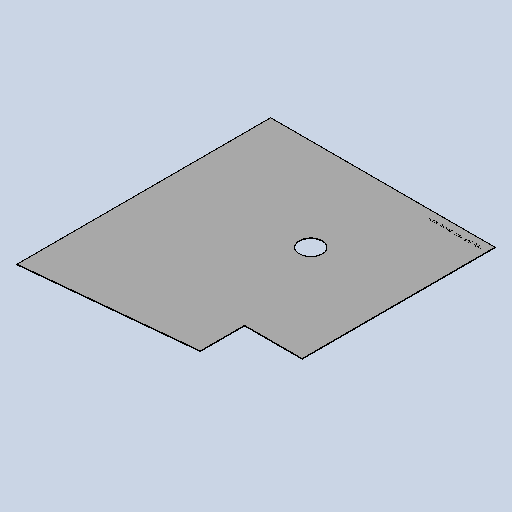
# Autodesk Inventor part: TRM 016 right board main+
Saved by Autodesk Inventor 2025 (Build 290162010, 162A)
## iProperties
Created: 2024-08-07
Part Number: TRM 016 right board main+
Material: AISI 304
Document SubType Name: Sheet Metal
Designer: pokla
Stock Number: ТРМ 015 левый борт основное
Density: 8.02768 g/cm^3
Flat Pattern Width: 77.93 cm
Flat Pattern Length: 88.1266 cm
Flat Pattern Area: 6867.71 cm^2
Sheet Metal Rule: AISI304 2mm Die16
Sheet Metal Width: 779,300 mm
Sheet Metal Length: 881,266 mm
Sheet Metal Area: 686770,668 mm^2
Appearance: Default
Author: pokla
Autodesk Inventor part; units mm, degrees
ref_plane "YZ Plane" through (0, 0, 0) normal (1, 0, 0) x (0, 1, 0)
ref_plane "XZ Plane" through (0, 0, 0) normal (0, 1, 0) x (-1, 0, 0)
ref_plane "XY Plane" through (0, 0, 0) normal (0, 0, 1) x (1, 0, 0)
sketch "Sketch1" plane through (0, 0, 0) normal (0, 0, 1) x (1, 0, 0)
  line L0 (-459.3004, -153.7378) -> (320, -153.7378)
  line L1 (320, -153.7378) -> (320, 670)
  line L2 (320, 670) -> (-459.3004, 670)
  line L3 (-459.3004, 670) -> (-459.3004, -153.7378)
  line L4 (120, -153.7378) -> (320, 0)
  circle A0 centre (0, 350) radius 40
  line L5 (320, 0) -> (120, 0)
  line L6 (120, 0) -> (120, -153.7378)
  line L7 (-459.3004, -153.7378) -> (-459.3004, -211.2657)
  line L8 (-459.3004, -211.2657) -> (120, -153.7378)
  point P0 (0, 0)
  dimension "d14" = 80
  dimension "d15" = 320
  dimension "d16" = 200
  dimension "d17" = 320
  dimension "d18" = 350
  measures "d14" diameter of A0
  measures "d15" distance from line of A0.centre L2
  measures "d16" distance of L4.end L5.end
  measures "d17" distance from line of L1 A0.centre
  measures "d18" distance of point (0, 0) A0.centre
extrude "Plate1" add sketch "Sketch1" along normal blind 2 contours L3 L2 L1 L5 L6 L0 | L0 L8 L7
sketch "Sketch2" plane through (0, 0, 0) normal (0, 0, -1) x (-1, 0, 0)
  line L0 (-300, 650) -> (-100, 650) construction
  line L1 (-100, 650) -> (-100, 630) construction
  line L2 (-100, 630) -> (-300, 630) construction
  line L3 (-300, 630) -> (-300, 650) construction
  line L4 (-320, 670) -> (459.3004, 670) projected
  line L5 (-320, 0) -> (-320, 670) projected
  point P0 (0, 0)
  point P1 (-48, 100)
  point P2 (459.3004, 670)
  point P3 (-251, -525)
  point P4 (-50, 98)
  dimension "d6" = 200
  dimension "d9" = 20
  dimension "d10" = 20
  dimension "d11" = 20
  constraints: 4 other
  measures "d6" distance of L0.start L0.end
  measures "d9" distance of L0.end L1.end
  measures "d11" length of L3
mark "Mark1"
equation "\"d2\" = Thickness"
equation "\"BendReliefWidth\" = Thickness"
equation "\"BendReliefDepth\" = 0.5 * Thickness"
equation "\"CornerReliefSize\" = 4 * Thickness"
equation "\"MinimumRemnant\" = 2 * Thickness"
equation "\"TransitionRadius\" = BendRadius"
equation "\"JacobiRadiusSize\" = BendRadius"
equation "\"GapSize\" = Thickness"
equation "\"Thickness\" = 2"
equation "\"BendRadius\" = 2.75"
body "Solid1"
